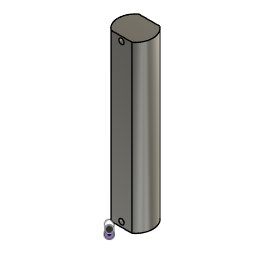
持ち手 v1 (Autodesk Fusion 360 design; units mm, degrees)
Autodesk Fusion 360 part; units mm, degrees
sketch "スケッチ1" plane through (0, 0, 0) normal (0, 0, 1) x (1, 0, 0)
  circle A0 centre (0, 0) radius 10
  dimension "d1" = 20
  constraint coincident A0.centre origin
  measures "d1" diameter of A0
extrude "押し出し1" add sketch "スケッチ1" along normal blind 95
sketch "スケッチ2" plane through (0, 0, 0) normal (1, 0, 0) x (0, 1, 0)
  line L0 (0, 0) -> (0, 5)
  line L1 (0, 0) -> (0, 2.5)
  circle A0 centre (0, 2.5) radius 1.5
  dimension "d4" = 3
  constraint coincident L0.start L1.start
  constraint vertical L0
  constraint midpoint L0 L1.end
  constraint coincident L1.end A0.centre
  measures "d4" diameter of A0
move_body "移動1" bodies 1 to x (1, 0, 0) y (0, 1, 0) z (0, 0, 1) at (0, 15, 0)
sketch "スケッチ3" plane through (0, 0, 0) normal (0, 0, 1) x (1, 0, 0)
  line L0 (6, 7) -> (-6, 7)
  line L1 (-6, 7) -> (-6, 5)
  line L2 (6, 7) -> (-6, 7)
  line L3 (-6, 7) -> (-6, 4.5)
  line L4 (-6, 4.5) -> (6, 4.5)
  line L5 (6, 4.5) -> (6, 7)
  constraint horizontal L0
  constraint perpendicular L0 L1
  constraint horizontal L2
  constraint vertical L3
  constraint horizontal L4
  constraint vertical L5
extrude "押し出し2" cut sketch "スケッチ3" along normal blind 100
sketch "スケッチ4" plane through (0, 0, 0) normal (0, 1, 0) x (1, 0, 0)
  line L0 (0, 0) -> (0, -0.2591)
  line L1 (0, -0.2591) -> (0, -2.7591)
  line L2 (0, -95) -> (0, -92.5)
  circle A0 centre (0, -92.5) radius 1.5
  circle A1 centre (0, -2.7591) radius 1.5
  dimension "d7" = 2.5
  dimension "d8" = 2.5
  dimension "d9" = 3
  dimension "d10" = 3
  constraint coincident L0.start origin
  constraint vertical L0
  constraint parallel L0 L1
  constraint vertical L2
  constraint coincident L2.end A0.centre
  constraint coincident L1.end A1.centre
  measures "d7" distance of L0.end L1.end
  measures "d8" distance of L2.start L2.end
  measures "d9" diameter of A0
  measures "d10" diameter of A1
extrude "押し出し3" cut sketch "スケッチ4" along normal blind 50
sketch "スケッチ5" plane through (0, 0, 0) normal (0, 0, 1) x (1, 0, 0)
  line L0 (-6, 23) -> (6, 23)
  line L1 (6, 23) -> (6, 26)
  line L2 (6, 26) -> (-6, 26)
  line L3 (-6, 26) -> (-6, 23)
  constraint horizontal L0
  constraint vertical L1
  constraint horizontal L2
  constraint vertical L3
extrude "押し出し4" cut sketch "スケッチ5" along normal blind 100
sketch "スケッチ6" plane through (0, 0, 0) normal (0, 0, 1) x (1, 0, 0)
